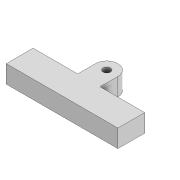
# Autodesk Inventor part: Fix_pin
Saved by Autodesk Inventor 2022 (Build 260153000, 153)
## iProperties
Created: 2022-04-23
Part Number: Fix_pin
Material: Generic
Document SubType Name: Modeling
Designer: dell
Density: 1 g/cm^3
Appearance: Default
Author: dell
Autodesk Inventor part; units mm, degrees
ref_plane "YZ Plane" through (0, 0, 0) normal (1, 0, 0) x (0, 1, 0)
ref_plane "XZ Plane" through (0, 0, 0) normal (0, 1, 0) x (-1, 0, 0)
ref_plane "XY Plane" through (0, 0, 0) normal (0, 0, 1) x (1, 0, 0)
sketch "Sketch1" plane through (0, 0, 0) normal (0, 1, 0) x (-1, 0, 0)
  circle A0 centre (0, 0) radius 1.65
  line L0 (5, -5) -> (-5, -5)
  line L1 (-5, -5) -> (-5, 20)
  line L2 (-5, 20) -> (5, 20)
  line L3 (5, 20) -> (5, -5)
  circle A1 centre (0, 0) radius 5
  line L4 (25, 8) -> (-25, 8)
  line L5 (-25, 8) -> (-25, 20)
  line L6 (-25, 20) -> (25, 20)
  line L7 (25, 20) -> (25, 8)
  point P0 (-5, 0)
  point P1 (5, 0)
  point P2 (5, 8)
  point P3 (-5, 8)
  dimension "d0" = 3.3
  dimension "d1" = 10
  dimension "d2" = 20
  dimension "d5" = 12
  dimension "d6" = 20
  dimension "d7" = 20
  constraints: 16 end point, 4 parallel, 3 tangent, 2 centre point, 2 coincident, 2 horizontal, 2 perpendicular, 1 collinear
  measures "d0" diameter of A0
  measures "d1" diameter of A1
  measures "d2" distance from line of point (0, 0) L2
  measures "d5" distance between parallel lines of L4 L2
  measures "d6" distance between parallel lines of L3 L7
  measures "d7" distance between parallel lines of L5 L1
extrude "Extrusion1" add sketch "Sketch1" along normal blind 8 contours A1 | A1 L1 L4 L3 | L4 L1 L2 L3 | L3 L6 L7 L4 | L4 L5 L6 L1
body "Solid1"
